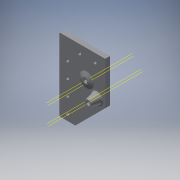
# Autodesk Inventor part: bracket-GT2-right
Saved by Autodesk Inventor 2018 (Build 220112000, 112)
## iProperties
Created: 2017-10-07
Part Number: bracket-GT2-right
Material: Generic
Document SubType Name: Modeling
Designer: Jurjen
Density: 1 g/cm^3
Appearance: Default
Author: Jurjen
Autodesk Inventor part; units mm, degrees
ref_plane "YZ Plane" through (0, 0, 0) normal (1, 0, 0) x (0, 1, 0)
ref_plane "XZ Plane" through (0, 0, 0) normal (0, 1, 0) x (-1, 0, 0)
ref_plane "XY Plane" through (0, 0, 0) normal (0, 0, 1) x (1, 0, 0)
sketch "Sketch1" plane through (0, 0, 0) normal (0, 0, 1) x (1, 0, 0)
  line L0 (-45, 45) -> (-45, -45)
  line L1 (-45, -45) -> (-25, -45)
  line L2 (-25, -45) -> (45, 25)
  line L3 (45, 25) -> (45, 45)
  line L4 (45, 45) -> (-45, 45)
  point P0 (0, 0)
  point P1 (0, 45)
  point P2 (-45, 0)
  dimension "d0" = 20
  dimension "d1" = 20
  dimension "d2" = 90
  dimension "d3" = 90
  constraints: 10 end point, 2 midpoint, 2 perpendicular, 1 horizontal alignment, 1 parallel, 1 vertical, 1 vertical alignment
  measures "d0" distance of L2.end L3.end
  measures "d1" distance of L0.end L1.end
  measures "d2" distance of L3.end L0.start
  measures "d3" distance of L0.start L0.end
extrude "Extrusion1" add sketch "Sketch1" along normal blind 6
sketch "Sketch2" plane through (0, 0, 6) normal (0, 0, 1) x (1, 0, 0)
  circle A0 centre (-11, 11) radius 2.5
  circle A1 centre (2, -2) radius 2.5
  line L0 (-25, -45) -> (45, 25) projected
  line L1 (45, 45) -> (-45, 45) projected
  line L2 (10, -10) -> (-45, 45) construction
  line L3 (-45, 45) -> (-45, -45) projected
  point P0 (0, 0)
  dimension "d6" = 5
  dimension "d7" = 34
  dimension "d8" = 13
  constraints: 2 centre point, 2 end point, 2 point on line, 1 equal radius, 1 midpoint
  measures "d6" diameter of A1
  measures "d7" distance from line of L3 A0.centre
  measures "d8" horizontal distance of A1.centre A0.centre
extrude "Extrusion2" cut sketch "Sketch2" against normal blind 6
ref_plane "Work Plane2" through (-11, 11, 6) normal (0.7071068, -0.7071068, 0) x (0.7071068, 0.7071068, 0)
ref_plane "Work Plane1" through (-9.2322, 9.2322, 6) normal (0.7071068, -0.7071068, 0) x (0.7071068, 0.7071068, 0)
sketch "Sketch3" plane through (-11, 11, 6) normal (0.7071068, -0.7071068, 0) x (0.7071068, 0.7071068, 0)
  line L0 (-49.4975, 0) -> (49.4975, 0) projected
  line L1 (0, 2) -> (0, 0)
  line L2 (-9, 0) -> (0, 0)
  line L3 (-9, 0) -> (-4, 2)
  line L4 (-4, 2) -> (0, 2)
  point P0 (0, -6)
  dimension "d12" = 9
  dimension "d13" = 2
  dimension "d17" = 4
  constraints: 8 end point, 1 horizontal, 1 midpoint, 1 perpendicular, 1 point on line
  measures "d12" distance of L2.start L1.end
  measures "d13" distance of L1.start L1.end
  measures "d17" distance of L3.end L1.start
revolve "Revolution1" add sketch "Sketch3" angle 360 about axis through (-11, 11, 8) along (0, 0, -1)
sketch "Sketch4" plane through (-11, 11, 6) normal (0, 0, -1) x (-1, 0, 0)
  circle A0 centre (0, 0) radius 2.5 projected
  point P0 (-11, -11)
extrude "Extrusion3" cut sketch "Sketch4" against normal up to next
sketch "Sketch5" plane through (0, 0, 6) normal (0, 0, 1) x (1, 0, 0)
  circle A0 centre (-35, -37) radius 2.1
  circle A1 centre (-35, -18) radius 2.1
  circle A2 centre (-35, 20) radius 2.1
  circle A3 centre (-20, 35) radius 2.1
  circle A4 centre (-1, 35) radius 2.1
  circle A5 centre (18, 35) radius 2.1
  circle A6 centre (37, 35) radius 2.1
  line L0 (-45, -45) -> (-25, -45) projected
  line L1 (45, 25) -> (45, 45) projected
  circle A7 centre (-35, 1) radius 2.1
  point P0 (0, 0)
  point P1 (45, 35)
  point P2 (-35, -45)
  point P3 (-35, -45)
  point P4 (-35, -45)
  dimension "d18" = 4.2
  dimension "d19" = 8
  dimension "d20" = 19
  dimension "d21" = 19
  dimension "d22" = 19
  dimension "d23" = 8
  dimension "d24" = 19
  dimension "d25" = 19
  dimension "d26" = 19
  constraints: 8 centre point, 7 equal radius, 5 vertical alignment, 4 horizontal alignment, 4 midpoint
  measures "d18" diameter of A0
  measures "d19" distance of A0.centre point (-35, -45)
  measures "d20" distance of A1.centre A0.centre
  measures "d21" distance of A7.centre A1.centre
  measures "d22" distance of A2.centre A7.centre
  measures "d23" distance of A6.centre point (45, 35)
  measures "d24" distance of A6.centre A5.centre
  measures "d25" distance of A4.centre A5.centre
  measures "d26" distance of A4.centre A3.centre
extrude "Extrusion4" cut sketch "Sketch5" against normal up to next
sketch "Sketch7" plane through (0, 0, 0) normal (0, 0, -1) x (-1, 0, 0)
  line L0 (15.5, 13.5239) -> (15.5, 8.4761)
  line L1 (15.5, 8.4761) -> (11, 5.7264)
  line L2 (11, 5.7264) -> (6.5, 8.4761)
  line L3 (6.5, 8.4761) -> (6.5, 13.5239)
  line L4 (6.5, 13.5239) -> (11, 16.2736)
  line L5 (11, 16.2736) -> (15.5, 13.5239)
  circle A0 centre (11, 11) radius 2.5 projected
  circle A1 centre (11, 11) radius 4.5 construction
  point P0 (0, 0)
  point P1 (15.5, 11)
  dimension "d30" = 9
  dimension "d32" = 9
  constraints: 12 end point, 3 horizontal alignment, 3 parallel, 2 vertical alignment, 1 centre point, 1 coincident, 1 midpoint, 1 tangent, 1 vertical
  measures "d30" distance between parallel lines of L3 L0
  measures "d32" distance between parallel lines of L1 L4
extrude "Extrusion5" cut sketch "Sketch7" against normal blind 5
ref_plane "Work Plane4" through (2, -2, 6) normal (0.7071068, -0.7071068, 0) x (0.7071068, 0.7071068, 0)
ref_plane "Work Plane3" through (0.2322, -0.2322, 6) normal (0.7071068, -0.7071068, 0) x (0.7071068, 0.7071068, 0)
sketch "Sketch8" plane through (2, -2, 6) normal (0.7071068, -0.7071068, 0) x (0.7071068, 0.7071068, 0)
  line L0 (2.5, -6) -> (-2.5, -6) projected
  line L1 (-2.5, 0) -> (2.5, 0) projected
  line L2 (-2.5, 0) -> (2.5, 0) projected
  line L3 (-2.5, 0) -> (-6.5, 0)
  line L4 (-6.5, 0) -> (-4, 11.5)
  line L5 (-4, 11.5) -> (-2.5, 11.5)
  line L6 (-2.5, 0) -> (-2.5, 11.5)
  line L7 (0, 0) -> (0, 4.1579) construction
  point P0 (0, -6)
  dimension "d36" = 4
  dimension "d37" = 1.5
  dimension "d38" = 11.5
  constraints: 10 end point, 1 midpoint, 1 parallel, 1 perpendicular, 1 point on line, 1 vertical
  measures "d36" distance of L1.start L3.end
  measures "d37" distance of L4.end L5.end
  measures "d38" distance of L1.start L5.end
revolve "Revolution2" add sketch "Sketch8" angle 360 about axis through (2, -2, 6) along (0, 0, 1)
fillet "Fillet2" radius 2 1 edges at (6.5962, 2.5962, 6)
fillet "Fillet3" radius 2 5 edges at (-45, -45, 3) (-25, -45, 3) (45, 25, 3) (45, 45, 3) (-45, 45, 3)
sketch "Sketch9" plane through (0, 0, 6) normal (0, 0, 1) x (1, 0, 0)
  line L0 (45, 60.6981) -> (12, 60.6981)
  line L1 (12, 60.6981) -> (12, -8.5167)
  line L2 (12, -8.5167) -> (45, -8.5167)
  line L3 (45, -8.5167) -> (45, 60.6981)
  point P0 (0, 0)
  point P1 (45, 43)
  dimension "d42" = 33
  constraints: 8 end point, 2 parallel, 1 horizontal, 1 perpendicular, 1 vertical alignment
  measures "d42" distance between parallel lines of L1 L3
extrude "Extrusion6" cut sketch "Sketch9" against normal up to next
equation "\"d21\" = d20"
equation "\"d22\" = d20"
equation "\"d23\" = d19"
equation "\"d24\" = d20"
equation "\"d25\" = d20"
equation "\"d26\" = d20"
body "Solid1"
